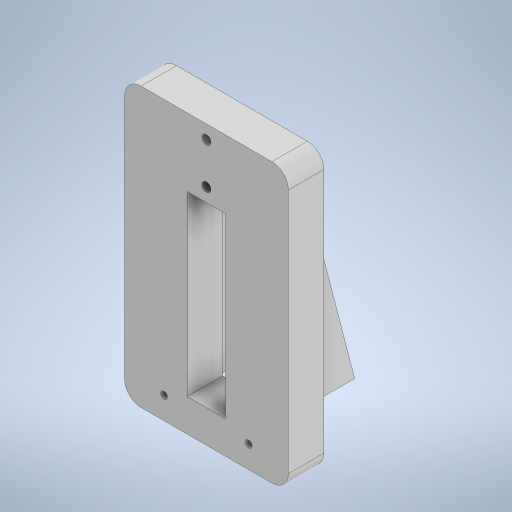
# Autodesk Inventor part: stand_less_rough
Saved by Autodesk Inventor 2024 (Build 280153000, 153)
## iProperties
Created: 2023-03-06
Part Number: stand_less_rough
Material: Generic
Document SubType Name: Modeling
Designer: frane
Density: 1 g/cm^3
Appearance: Default
Author: frane
Autodesk Inventor part; units mm, degrees
ref_plane "YZ Plane" through (0, 0, 0) normal (1, 0, 0) x (0, 1, 0)
sketch "Sketch1" plane through (0, 0, 0) normal (0, 0, 1) x (1, 0, 0)
  line L0 (0, 0) -> (-60, 0)
  line L1 (-60, 0) -> (-60, 20)
  line L2 (-60, 20) -> (-60, 110)
  line L3 (-60, 110) -> (-30, 110)
  line L4 (-30, 0) -> (-30, 110)
  line L5 (-30, 20) -> (-55.65, 20)
  line L6 (-55.65, 20) -> (-55.65, 85)
  line L7 (-55.65, 85) -> (-30, 85)
  line L8 (0, 20) -> (0, 110)
  line L9 (0, 110) -> (-30, 110)
  line L10 (-30, 20) -> (-4.35, 20)
  line L11 (-4.35, 20) -> (-4.35, 85)
  line L12 (-4.35, 85) -> (-30, 85)
  line L13 (0, 0) -> (0, 20)
  line L14 (-30, 20) -> (-45, 20)
  dimension "d0" = 60
  dimension "d1" = 20
  dimension "d2" = 90
  dimension "d3" = 65
  dimension "d39" = 15
  constraints: 30 end point, 6 perpendicular, 4 point on line, 4 symmetric about line, 2 horizontal, 1 midpoint, 1 vertical
  measures "d0" distance of L0.start L0.end
  measures "d1" distance of L0.end L1.end
  measures "d2" distance of L1.end L2.end
  measures "d3" distance of L5.end L6.end
  measures "d39" distance of L5.start L14.end
extrude "Extrusion1" add sketch "Sketch1" along normal mid plane 13 contours L0 L4 L10 L11 L12 L9 L8 L13 | L0 L1 L2 L3 L4 L7 L6 L5
sketch "Sketch2" plane through (0, 0, 6.5) normal (1, 0, 0) x (0, 0, -1)
  line L0 (13, 0) -> (13, 110) projected
  line L1 (13, 0) -> (13, 20)
  line L2 (13, 20) -> (36.3, 20)
  line L3 (36.3, 20) -> (13, 110)
  point P0 (6.5, 0)
  dimension "d6" = 20
  dimension "d7" = 23.3
  constraints: 6 end point, 1 perpendicular, 1 point on line
  measures "d6" distance of L0.start L1.end
  measures "d7" distance of L1.end L2.end
extrude "Extrusion2" add sketch "Sketch2" against normal blind 22
ref_plane "Work Plane1" through (-30, 20, 6.5) normal (-1, 0, 0) x (0, 0, 1)
mirror "Mirror1" about plane through (-30, 20, 6.5) normal (-1, 0, 0) of "Extrusion2"
sketch "Sketch3" plane through (0, 0, 6.5) normal (0, 0, 1) x (1, 0, 0)
  line L0 (-4.35, 20) -> (-55.65, 20) projected
  line L1 (-30, 20) -> (-30, 0)
  line L2 (-60, 0) -> (0, 0) projected
  line L3 (-30, 16.1731) -> (-45.5, 16.1731)
  line L4 (-30, 16.1731) -> (-14.5, 16.1731)
  dimension "d17" = 15.5
  constraints: 6 end point, 2 coincident, 2 midpoint, 1 perpendicular, 1 point on line, 1 symmetric about line
  measures "d17" distance of L3.start L3.end
sketch "Sketch4" plane through (0, 0, 6.5) normal (0, 0, 1) x (1, 0, 0)
  line L0 (-55.65, 85) -> (-4.35, 85) projected
  line L1 (-30, 85) -> (-30, 110)
  line L2 (0, 110) -> (-60, 110) projected
  line L3 (-30, 85) -> (-30, 90)
  line L4 (-30, 90) -> (-30, 105)
  point P0 (0, 0)
  dimension "d25" = 5
  dimension "d26" = 15
  constraints: 6 end point, 2 coincident, 2 midpoint, 2 point on line
  measures "d25" distance of L1.start L3.end
  measures "d26" distance of L3.end L4.end
hole "Hole2" at (-30, 90, 6.5) at (-30, 105, 6.5) direction (0, 0, -1) diameter 3.242 end through all thread size "M4x0.7" class "6H" standard "ISO Metric profile"
sketch "Sketch5" plane through (-60, 20, -29.8) normal (0, -1, 0) x (1, 0, 0)
  line L0 (0, 0) -> (22, 0) projected
  line L1 (0, 0) -> (0, 6)
  line L2 (0, 0) -> (0, 23.3) projected
  line L3 (0, 6) -> (60, 6)
  line L4 (60, 0) -> (60, 23.3) projected
  line L5 (60, 6) -> (43, 6)
  line L6 (0, 6) -> (17, 6)
  point P0 (60, 29.8)
  point P1 (17, 6)
  dimension "d34" = 6
  dimension "d35" = 17
  dimension "d36" = 17
  constraints: 8 end point, 4 point on line, 2 coincident, 1 perpendicular
  measures "d34" distance of L0.start L1.end
  measures "d35" distance of L3.end L5.end
  measures "d36" distance of L1.end L6.end
hole "Hole3" at (-43, 20, -23.8) at (-17, 20, -23.8) direction (0, 1, 0) diameter 3 end through all
sketch "Sketch6" plane through (0, 0, 6.5) normal (1, 0, 0) x (0, 0, -1)
  line L0 (13, 110) -> (0, 110) projected
  line L1 (13, 0) -> (13, 20) projected
  line L2 (13, 110) -> (13, 20)
  line L3 (36.3, 20) -> (13, 20) projected
  line L4 (13, 20) -> (36.3, 20)
  line L5 (13, 110) -> (36.3, 20) projected
  line L6 (36.3, 20) -> (13, 110)
  point P0 (6.5, 0)
  constraints: 6 end point, 2 collinear, 1 vertical
extrude "Extrusion3" cut sketch "Sketch6" against normal blind 12
mirror "Mirror2" about plane through (-30, 20, 6.5) normal (-1, 0, 0) of "Extrusion3"
sketch "Sketch8" plane through (0, 0, 6.5) normal (0, 0, 1) x (1, 0, 0)
  line L0 (-4.35, 20) -> (-55.65, 20) projected
  line L1 (-30, 20) -> (-30, 85)
  line L2 (-55.65, 85) -> (-4.35, 85) projected
  line L3 (-30, 20) -> (-37, 20)
  line L4 (-37, 20) -> (-37, 85)
  line L5 (-55.65, 20) -> (-55.65, 85) projected
  line L6 (-37, 85) -> (-55.65, 85)
  line L7 (-55.65, 85) -> (-55.65, 20)
  line L8 (-55.65, 20) -> (-37, 20)
  line L9 (-23, 20) -> (-23, 85)
  line L10 (-4.35, 20) -> (-4.35, 85)
  line L11 (-23, 85) -> (-4.35, 85)
  line L12 (-4.35, 85) -> (-4.35, 20)
  line L13 (-4.35, 20) -> (-23, 20)
  point P0 (0, 0)
  point P1 (-23, 85)
  dimension "d43" = 7
  constraints: 22 end point, 5 perpendicular, 2 midpoint, 2 symmetric about line
  measures "d43" distance of L1.start L3.end
extrude "Extrusion5" add sketch "Sketch8" against normal blind 13 contours L0 L9 L2 L10 | L0 L5 L2 L4
sketch "Sketch9" plane through (-60, 0, 6.5) normal (0, -1, 0) x (1, 0, 0)
  line L0 (60, -13) -> (60, 0) projected
  line L1 (60, 0) -> (0, 0) projected
  line L2 (60, -13) -> (0, -13)
  line L3 (0, -13) -> (0, 0)
  line L4 (0, 0) -> (60, 0)
  line L5 (60, 0) -> (60, -13)
  point P0 (60, -6.5)
  constraints: 8 end point, 2 parallel, 1 horizontal, 1 perpendicular
extrude "Extrusion6" cut sketch "Sketch9" against normal blind 8
fillet "Fillet1" radius 6 4 edges at (0, 8, 0) (-60, 8, 0) (-60, 110, 0) (0, 110, 0)
fillet "Fillet2" radius 4 2 edges at (-48, 65, -6.5) (-12, 65, -6.5)
ref_plane "Work Plane2" through (-54, 110, 6.5) normal (0, 1, 0) x (1, 0, 0)
sketch "Sketch10" plane through (-54, 110, 6.5) normal (0, 1, 0) x (1, 0, 0)
  circle A0 centre (11, 30.3) radius 1.5 projected
  line L0 (11, 30.3) -> (11, 36.3)
  line L1 (6, 36.3) -> (16, 36.3) projected
  circle A1 centre (37, 30.3) radius 1.5 projected
  line L2 (37, 30.3) -> (37, 36.3)
  line L3 (42, 36.3) -> (32, 36.3) projected
  point P0 (54, 6.5)
  constraints: 4 end point, 2 coincident, 2 midpoint
hole "Hole4" at (-43, 110, -23.8) at (-17, 110, -23.8) direction (0, -1, 0) diameter 7 depth 85
hole "Hole5" at (-14.5, 16.1731, 6.5) at (-45.5, 16.1731, 6.5) direction (0, 0, -1) diameter 2.4 end through all clearance for "Countersunk Flat Head Screw ISO 2009/7046" size "M2" standard "ISO"
thread "Thread1" size "M5x0.8" class "6H" standard "ISO Metric profile" full length
thread "Thread2" size "M5x0.8" class "6H" standard "ISO Metric profile" full length
body "Solid1"
